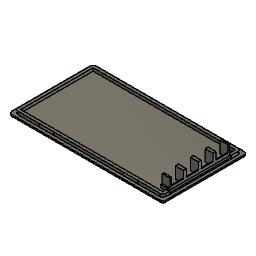
ROC_rev_C+_bottom (Autodesk Fusion 360 design; units mm, degrees)
Autodesk Fusion 360 part; units mm, degrees
sketch "Sketch11" plane through (0, 16, 0) normal (0, -1, 0) x (1, 0, 0)
  line L0 (26.9, -42.9) -> (26.9, -57.9)
  arc A0 (24.9, -59.9) -> (26.9, -57.9) centre (24.9, -57.9) ccw
  line L1 (24.9, -59.9) -> (-24.9, -59.9)
  arc A1 (-26.9, -57.9) -> (-24.9, -59.9) centre (-24.9, -57.9) ccw
  line L2 (-26.9, -57.9) -> (-26.9, -42.9)
  line L3 (-26.9, -42.9) -> (-26.9, -32.9)
  line L4 (-26.9, -32.9) -> (-26.9, 14.9)
  line L5 (-26.9, 14.9) -> (-26.9, 24.9)
  line L6 (-26.9, 24.9) -> (-26.9, 39.9)
  arc A2 (-24.9, 41.9) -> (-26.9, 39.9) centre (-24.9, 39.9) ccw
  line L7 (-24.9, 41.9) -> (24.9, 41.9)
  arc A3 (26.9, 39.9) -> (24.9, 41.9) centre (24.9, 39.9) ccw
  line L8 (26.9, 39.9) -> (26.9, 24.9)
  line L9 (26.9, 24.9) -> (26.9, 14.9)
  line L10 (26.9, 14.9) -> (26.9, -32.9)
  line L11 (26.9, -32.9) -> (26.9, -42.9)
  arc A4 (29, 42) -> (27, 44) centre (27, 42) ccw
  line L12 (27, 44) -> (-27, 44)
  arc A5 (-27, 44) -> (-29, 42) centre (-27, 42) ccw
  line L13 (-29, 42) -> (-29, -60)
  arc A6 (-29, -60) -> (-27, -62) centre (-27, -60) ccw
  line L14 (-27, -62) -> (27, -62)
  arc A7 (27, -62) -> (29, -60) centre (27, -60) ccw
  line L15 (29, -60) -> (29, 42)
  line L16 (-26.9, -32.9) -> (-29, -32.9)
  line L17 (-29, -32.9) -> (-29, -42.9)
  line L18 (-29, -42.9) -> (-26.9, -42.9)
  line L19 (-26.9, -42.9) -> (-26.9, -32.9)
  line L20 (-26.9, 24.9) -> (-29, 24.9)
  line L21 (-29, 24.9) -> (-29, 14.9)
  line L22 (-29, 14.9) -> (-26.9, 14.9)
  line L23 (-26.9, 14.9) -> (-26.9, 24.9)
  line L24 (26.9, 24.9) -> (29, 24.9)
  line L25 (29, 24.9) -> (29, 14.9)
  line L26 (29, 14.9) -> (26.9, 14.9)
  line L27 (26.9, 14.9) -> (26.9, 24.9)
  line L28 (26.9, -32.9) -> (29, -32.9)
  line L29 (29, -32.9) -> (29, -42.9)
  line L30 (29, -42.9) -> (26.9, -42.9)
  line L31 (26.9, -42.9) -> (26.9, -32.9)
  dimension "d1" = 10
  dimension "d2" = 2.1
  dimension "d3" = 10
  dimension "d4" = 10
  dimension "d5" = 10
  constraint horizontal L16
  constraint vertical L17
  constraint horizontal L18
  constraint vertical L19
  constraint coincident L3.end L4.start
  constraint horizontal L20
  constraint vertical L21
  constraint horizontal L22
  constraint vertical L23
  constraint coincident L5.end L6.start
  constraint horizontal L24
  constraint vertical L25
  constraint horizontal L26
  constraint vertical L27
  constraint coincident L8.end L9.start
  constraint horizontal L28
  constraint vertical L29
  constraint horizontal L30
  constraint vertical L31
  constraint coincident L10.end L11.start
  measures "d1" distance of L3.end L2.end
  measures "d2" distance of L5.end L20.end
  measures "d3" distance of L5.end L4.end
  measures "d4" distance of L8.end L9.end
  measures "d5" distance of L10.end L0.start
sketch "Sketch2" plane through (0, 0, 0) normal (0, 1, 0) x (1, 0, 0)
  line L0 (51, -29) -> (-51, -29)
  line L1 (-53, -27) -> (-53, 27)
  line L2 (-51, 29) -> (51, 29)
  line L3 (53, 27) -> (53, -27)
  line L4 (53, -29) -> (-53, 29) construction
  line L5 (-53, -29) -> (53, 29) construction
  arc A0 (-51, 29) -> (-53, 27) centre (-51, 27) ccw
  arc A1 (53, 27) -> (51, 29) centre (51, 27) ccw
  arc A2 (51, -29) -> (53, -27) centre (51, -27) ccw
  arc A3 (-53, -27) -> (-51, -29) centre (-51, -27) ccw
  dimension "d255" = 106
  dimension "d256" = 58
  dimension "d257" = 2
  dimension "d265" = 0
  dimension "d266" = 0
  dimension "d267" = 0
  dimension "d268" = 0
  constraint perpendicular L0 L1
  constraint parallel L0 L2
  constraint parallel L1 L3
  constraint horizontal L0
  constraint coincident L4 origin
  constraint coincident L5 origin
  constraint coincident L4.end L1
  constraint coincident L4.end L2
  constraint tangent L1 A0
  constraint tangent L2 A0
  constraint coincident L5.end L2
  constraint coincident L5.end L3
  constraint tangent L2 A1
  constraint tangent L3 A1
  constraint equal A0 A1
  constraint coincident L4.start L3
  constraint coincident L4.start L0
  constraint tangent L3 A2
  constraint tangent L0 A2
  constraint equal A0 A2
  constraint coincident L5.start L0
  constraint coincident L5.start L1
  constraint tangent L0 A3
  constraint tangent L1 A3
  constraint equal A0 A3
  measures "d255" distance of L4.end L5.end
  measures "d256" distance of L5.start L4.end
  measures "d257" radius of A0
extrude "Extrude1" add sketch "Sketch2" along normal blind 2
sketch "Sketch3" plane through (0, 2, 0) normal (0, 1, 0) x (-1, 0, 0)
  arc A0 (51, -29) -> (53, -27) centre (51, -27) ccw
  line L0 (53, -27) -> (53, 27)
  arc A1 (53, 27) -> (51, 29) centre (51, 27) ccw
  line L1 (51, 29) -> (-51, 29)
  arc A2 (-51, 29) -> (-53, 27) centre (-51, 27) ccw
  line L2 (-53, 27) -> (-53, -27)
  arc A3 (-53, -27) -> (-51, -29) centre (-51, -27) ccw
  line L3 (-51, -29) -> (51, -29)
  line L4 (50.9, -24.9) -> (50.9, 24.9)
  line L5 (48.9, 26.9) -> (-48.9, 26.9)
  line L6 (-50.9, 24.9) -> (-50.9, -24.9)
  line L7 (-48.9, -26.9) -> (48.9, -26.9)
  arc A4 (48.9, -26.9) -> (50.9, -24.9) centre (48.9, -24.9) ccw
  arc A5 (-50.9, -24.9) -> (-48.9, -26.9) centre (-48.9, -24.9) ccw
  arc A6 (-48.9, 26.9) -> (-50.9, 24.9) centre (-48.9, 24.9) ccw
  arc A7 (50.9, 24.9) -> (48.9, 26.9) centre (48.9, 24.9) ccw
  line L8 (-48.9, 24.9) -> (-48.9, -24.9)
  line L9 (-48.9, -24.9) -> (48.9, -24.9)
  line L10 (48.9, -24.9) -> (48.9, 24.9)
  line L11 (48.9, 24.9) -> (-48.9, 24.9)
  dimension "d261" = 2
  dimension "d262" = -2
  dimension "d277" = 2.1
  dimension "d278" = 2.1
  dimension "d279" = 2.1
  dimension "d280" = 2.1
  constraint parallel L0 L4
  constraint parallel L1 L5
  constraint parallel L2 L6
  constraint parallel L3 L7
  constraint tangent L4 A4
  constraint tangent L7 A4
  constraint tangent L7 A5
  constraint tangent L6 A5
  constraint equal A4 A5
  constraint tangent L5 A6
  constraint tangent L6 A6
  constraint equal A4 A6
  constraint tangent L5 A7
  constraint tangent L4 A7
  constraint equal A4 A7
  measures "d261" radius of A4
  measures "d277" distance of L3 L7
  measures "d278" distance of L0 L4
  measures "d279" distance of L1 L5
  measures "d280" distance of L2 L6
extrude "Extrude2" add sketch "Sketch3" along normal blind 2 contours L4 L5 L6 L7 A4 A5 A6 A7
sketch "Sketch4" plane through (0, 0, 26.9) normal (0, 0, 1) x (1, 0, 0)
  line L0 (-48.9, 2) -> (48.9, 2)
  line L1 (48.9, 2) -> (48.9, 4)
  line L2 (48.9, 4) -> (-48.9, 4)
  line L3 (-48.9, 4) -> (-48.9, 2)
  line L4 (33.9, 4) -> (23.9, 4)
  line L5 (23.9, 4) -> (23.9, 2)
  line L6 (23.9, 2) -> (33.9, 2)
  line L7 (33.9, 2) -> (33.9, 4)
  line L8 (-23.9, 4) -> (-33.9, 4)
  line L9 (-33.9, 4) -> (-33.9, 2)
  line L10 (-33.9, 2) -> (-23.9, 2)
  line L11 (-23.9, 2) -> (-23.9, 4)
  dimension "d289" = 10
  dimension "d290" = 10
  dimension "d291" = 15
  dimension "d292" = 15
  constraint horizontal L4
  constraint vertical L5
  constraint horizontal L6
  constraint vertical L7
  constraint coincident L2 L4.start
  constraint horizontal L8
  constraint vertical L9
  constraint horizontal L10
  constraint vertical L11
  constraint coincident L2 L8.start
  measures "d289" distance of L4.start L4.end
  measures "d290" distance of L8.start L8.end
  measures "d291" distance of L3 L9
  measures "d292" distance of L1 L7
extrude "Extrude3" add sketch "Sketch4" along normal blind 1 contours L0 L2 L8 L9 L10 L11 | L0 L2 L4 L5 L6 L7
sketch "Sketch5" plane through (-33.9, 0, 0) normal (-1, 0, 0) x (0, 0, 1)
  line L0 (26.9, 4) -> (26.9, 2)
  line L1 (26.9, 2) -> (27.9, 2)
  line L2 (27.9, 2) -> (27.9, 4)
  line L3 (27.9, 4) -> (26.9, 4)
  line L4 (26.9, 4) -> (27.9, 3)
  line L5 (26.9, 2) -> (27.9, 3)
  constraint coincident L0.start L3.end
  constraint midpoint L2 L4.end
  constraint coincident L0.end L1.start
extrude "Extrude4" cut sketch "Sketch5" against normal up to surface (67.8 mm away) contours L2 L3 L4 | L1 L2 L5
sketch "Sketch6" plane through (0, 0, -26.9) normal (0, 0, -1) x (-1, 0, 0)
  line L0 (-48.9, 2) -> (48.9, 2)
  line L1 (48.9, 2) -> (48.9, 4)
  line L2 (48.9, 4) -> (-48.9, 4)
  line L3 (-48.9, 4) -> (-48.9, 2)
  line L4 (33.9, 4) -> (23.9, 4)
  line L5 (23.9, 4) -> (23.9, 2)
  line L6 (23.9, 2) -> (33.9, 2)
  line L7 (33.9, 2) -> (33.9, 4)
  line L8 (-23.9, 4) -> (-33.9, 4)
  line L9 (-33.9, 4) -> (-33.9, 2)
  line L10 (-33.9, 2) -> (-23.9, 2)
  line L11 (-23.9, 2) -> (-23.9, 4)
  dimension "d297" = 10
  dimension "d298" = 10
  dimension "d299" = 15
  dimension "d300" = 15
  constraint horizontal L4
  constraint vertical L5
  constraint horizontal L6
  constraint vertical L7
  constraint coincident L2 L4.start
  constraint horizontal L8
  constraint vertical L9
  constraint horizontal L10
  constraint vertical L11
  constraint coincident L2 L8.start
  measures "d297" distance of L4.start L4.end
  measures "d298" distance of L8.start L8.end
  measures "d299" distance of L1 L7
  measures "d300" distance of L3 L9
extrude "Extrude5" add sketch "Sketch6" along normal blind 1 contours L0 L2 L8 L9 L10 L11 | L0 L2 L4 L5 L6 L7
sketch "Sketch7" plane through (33.9, 0, 0) normal (1, 0, 0) x (0, 0, -1)
  line L0 (26.9, 4) -> (26.9, 2)
  line L1 (26.9, 2) -> (27.9, 2)
  line L2 (27.9, 2) -> (27.9, 4)
  line L3 (27.9, 4) -> (26.9, 4)
  line L4 (26.9, 4) -> (27.9, 3)
  line L5 (27.9, 3) -> (26.9, 2)
  constraint coincident L0.start L3.end
  constraint midpoint L2 L4.end
  constraint coincident L0.end L1.start
extrude "Extrude6" cut sketch "Sketch7" against normal up to surface (67.8 mm away) contours L2 L3 L4 | L1 L2 L5
extrude "Extrude7" cut sketch "Sketch11" against normal blind 1 contours L11 L15 L28 L29 L30 L31 | L9 L15 L24 L25 L26 L27 | L3 L13 L16 L17 L18 L19 | L5 L13 L20 L21 L22 L23
chamfer "Chamfer1" [no effect]
fillet "Fillet1" radius 0.1 4 edges at (-28.9, 3, 27.9) (28.9, 3, 27.9) (-28.9, 3, -27.9) (28.9, 3, -27.9)
fillet "Fillet2" radius 1 8 edges at (-52.4142, 0, 28.4142) (-53, 0, 0) (-52.4142, 0, -28.4142) (0, 0, -29) (52.4142, 0, -28.4142) (53, 0, 0) (52.4142, 0, 28.4142) (0, 0, 29)
sketch "Sketch8" plane through (0, 2, 0) normal (0, 1, 0) x (-1, 0, 0)
  line L0 (-48.9, 24.9) -> (-48.9, -24.9)
  line L1 (-48.9, -24.9) -> (48.9, -24.9)
  line L2 (48.9, -24.9) -> (48.9, 24.9)
  line L3 (48.9, 24.9) -> (-48.9, 24.9)
  line L4 (-48.9, 21.4) -> (-43.9, 21.4)
  line L5 (-43.9, 21.4) -> (-43.9, 19.4)
  line L6 (-43.9, 19.4) -> (-48.9, 19.4)
  line L7 (-48.9, 19.4) -> (-48.9, 21.4)
  line L8 (-48.9, 24.9) -> (48.9, 24.9)
  line L9 (-48.9, 11.2) -> (-43.9, 11.2)
  line L10 (-43.9, 11.2) -> (-43.9, 9.2)
  line L11 (-43.9, 9.2) -> (-48.9, 9.2)
  line L12 (-48.9, 9.2) -> (-48.9, 11.2)
  line L13 (-48.9, 1) -> (-43.9, 1)
  line L14 (-43.9, 1) -> (-43.9, -1)
  line L15 (-43.9, -1) -> (-48.9, -1)
  line L16 (-48.9, -1) -> (-48.9, 1)
  line L17 (-48.9, -9.2) -> (-43.9, -9.2)
  line L18 (-43.9, -9.2) -> (-43.9, -11.2)
  line L19 (-43.9, -11.2) -> (-48.9, -11.2)
  line L20 (-48.9, -11.2) -> (-48.9, -9.2)
  line L21 (-48.9, -19.4) -> (-43.9, -19.4)
  line L22 (-43.9, -19.4) -> (-43.9, -21.4)
  line L23 (-43.9, -21.4) -> (-48.9, -21.4)
  line L24 (-48.9, -21.4) -> (-48.9, -19.4)
  dimension "d281" = 0
  dimension "d282" = 0
  dimension "d283" = 0
  dimension "d284" = 0
  dimension "d368" = 5
  dimension "d369" = 2
  dimension "d370" = 3.5
  dimension "d375" = 2
  dimension "d376" = 5
  dimension "d377" = 8.2
  dimension "d378" = 2
  dimension "d379" = 5
  dimension "d380" = 5
  dimension "d381" = 2
  dimension "d382" = 8.2
  dimension "d383" = 8.2
  dimension "d384" = 5
  dimension "d385" = 2
  dimension "d386" = 8.2
  constraint horizontal L4
  constraint vertical L5
  constraint horizontal L6
  constraint vertical L7
  constraint coincident L0 L4.start
  constraint horizontal L9
  constraint vertical L10
  constraint horizontal L11
  constraint vertical L12
  constraint coincident L0 L9.start
  constraint horizontal L13
  constraint vertical L14
  constraint horizontal L15
  constraint vertical L16
  constraint coincident L0 L13.start
  constraint horizontal L17
  constraint vertical L18
  constraint horizontal L19
  constraint vertical L20
  constraint coincident L0 L17.start
  constraint horizontal L21
  constraint vertical L22
  constraint horizontal L23
  constraint vertical L24
  constraint coincident L0 L21.start
  measures "d368" distance of L4.start L4.end
  measures "d369" distance of L4.start L6.end
  measures "d370" distance of L4 L8
  measures "d375" distance of L9.start L11.end
  measures "d376" distance of L9.start L9.end
  measures "d377" distance of L6 L9
  measures "d378" distance of L13.start L15.end
  measures "d379" distance of L13.start L13.end
  measures "d380" distance of L17.start L17.end
  measures "d381" distance of L17.start L19.end
  measures "d382" distance of L11 L13
  measures "d383" distance of L15 L17
  measures "d384" distance of L21.start L21.end
  measures "d385" distance of L21.start L23.end
  measures "d386" distance of L19 L21
extrude "Extrude8" add sketch "Sketch8" along normal up to surface (2 mm away) contours L0 L4 L5 L6 L7 | L0 L9 L10 L11 L12 | L0 L21 L22 L23 L24 | L0 L13 L14 L15 L16 | L0 L17 L18 L19 L20
sketch "Sketch9" plane through (0, 4, 0) normal (0, 1, 0) x (-1, 0, 0)
  line L0 (-48.9, 24.9) -> (48.9, 24.9)
  line L1 (48.9, 24.9) -> (48.9, -24.9)
  line L2 (48.9, -24.9) -> (-48.9, -24.9)
  line L3 (-48.9, -24.9) -> (-48.9, -21.4)
  line L4 (-48.9, 19.4) -> (-43.9, 19.4)
  line L5 (-43.9, 19.4) -> (-43.9, 21.4)
  line L6 (-43.9, 21.4) -> (-48.9, 21.4)
  line L7 (-48.9, 21.4) -> (-48.9, 24.9)
  line L8 (-33.9, -26.9) -> (-23.9, -26.9)
  line L9 (-23.9, -26.9) -> (23.9, -26.9)
  line L10 (23.9, -26.9) -> (33.9, -26.9)
  line L11 (33.9, -26.9) -> (48.9, -26.9)
  arc A0 (48.9, -26.9) -> (50.9, -24.9) centre (48.9, -24.9) ccw
  line L12 (50.9, -24.9) -> (50.9, 24.9)
  arc A1 (50.9, 24.9) -> (48.9, 26.9) centre (48.9, 24.9) ccw
  line L13 (48.9, 26.9) -> (33.9, 26.9)
  line L14 (33.9, 26.9) -> (23.9, 26.9)
  line L15 (23.9, 26.9) -> (-23.9, 26.9)
  line L16 (-23.9, 26.9) -> (-33.9, 26.9)
  line L17 (-33.9, 26.9) -> (-48.9, 26.9)
  arc A2 (-48.9, 26.9) -> (-50.9, 24.9) centre (-48.9, 24.9) ccw
  line L18 (-50.9, 24.9) -> (-50.9, -24.9)
  arc A3 (-50.9, -24.9) -> (-48.9, -26.9) centre (-48.9, -24.9) ccw
  line L19 (-48.9, -26.9) -> (-33.9, -26.9)
  line L20 (-48.9, -21.4) -> (-43.9, -21.4)
  line L21 (-43.9, -21.4) -> (-43.9, -19.4)
  line L22 (-43.9, -19.4) -> (-48.9, -19.4)
  line L23 (-48.9, -19.4) -> (-48.9, -11.2)
  line L24 (-48.9, -11.2) -> (-43.9, -11.2)
  line L25 (-43.9, -11.2) -> (-43.9, -9.2)
  line L26 (-43.9, -9.2) -> (-48.9, -9.2)
  line L27 (-48.9, -9.2) -> (-48.9, -1)
  line L28 (-48.9, -1) -> (-43.9, -1)
  line L29 (-43.9, -1) -> (-43.9, 1)
  line L30 (-43.9, 1) -> (-48.9, 1)
  line L31 (-48.9, 1) -> (-48.9, 9.2)
  line L32 (-48.9, 9.2) -> (-43.9, 9.2)
  line L33 (-43.9, 9.2) -> (-43.9, 11.2)
  line L34 (-43.9, 11.2) -> (-48.9, 11.2)
  line L35 (-48.9, 11.2) -> (-48.9, 19.4)
  line L36 (-43.9, -9.2) -> (-50.9, -9.2)
  line L37 (-50.9, -9.2) -> (-50.9, -11.2)
  line L38 (-50.9, -11.2) -> (-43.9, -11.2)
  line L39 (-43.9, -11.2) -> (-43.9, -9.2)
  line L40 (-43.9, 1) -> (-50.9, 1)
  line L41 (-50.9, 1) -> (-50.9, -1)
  line L42 (-50.9, -1) -> (-43.9, -1)
  line L43 (-43.9, -1) -> (-43.9, 1)
  line L44 (-43.9, 11.2) -> (-50.9, 11.2)
  line L45 (-50.9, 11.2) -> (-50.9, 9.2)
  line L46 (-50.9, 9.2) -> (-43.9, 9.2)
  line L47 (-43.9, 9.2) -> (-43.9, 11.2)
  line L48 (-43.9, -19.4) -> (-50.9, -19.4)
  line L49 (-50.9, -19.4) -> (-50.9, -20.4)
  line L50 (-50.9, -20.4) -> (-43.9, -20.4)
  line L51 (-43.9, -20.4) -> (-43.9, -19.4)
  line L52 (-43.9, 19.4) -> (-50.9, 19.4)
  line L53 (-50.9, 19.4) -> (-50.9, 20.4)
  line L54 (-50.9, 20.4) -> (-43.9, 20.4)
  line L55 (-43.9, 20.4) -> (-43.9, 19.4)
  dimension "d389" = 7
  dimension "d390" = 2
  dimension "d393" = 7
  dimension "d394" = 2
  dimension "d397" = 7
  dimension "d398" = 2
  dimension "d401" = 7
  dimension "d402" = 1
  dimension "d403" = 1
  dimension "d404" = 7
  constraint horizontal L36
  constraint vertical L37
  constraint horizontal L38
  constraint vertical L39
  constraint coincident L25.end L26.start
  constraint horizontal L40
  constraint vertical L41
  constraint horizontal L42
  constraint vertical L43
  constraint coincident L29.end L30.start
  constraint horizontal L44
  constraint vertical L45
  constraint horizontal L46
  constraint vertical L47
  constraint coincident L33.end L34.start
  constraint horizontal L48
  constraint vertical L49
  constraint horizontal L50
  constraint vertical L51
  constraint coincident L21.end L22.start
  constraint horizontal L52
  constraint vertical L53
  constraint horizontal L54
  constraint vertical L55
  constraint coincident L4.end L5.start
  measures "d389" distance of L25.end L36.end
  measures "d390" distance of L25.end L24.end
  measures "d393" distance of L29.end L40.end
  measures "d394" distance of L29.end L28.end
  measures "d397" distance of L33.end L44.end
  measures "d398" distance of L33.end L32.end
  measures "d401" distance of L21.end L48.end
  measures "d402" distance of L21.end L50.end
  measures "d403" distance of L4.end L54.end
  measures "d404" distance of L4.end L52.end
extrude "Extrude9" add sketch "Sketch9" along normal blind 6 contours L4 L5 L18 L52 L53 L54 L55 | L18 L21 L22 L48 L49 L50 L51 | L18 L32 L33 L34 L44 L45 L46 L47 | L18 L28 L29 L30 L40 L41 L42 L43 | L18 L24 L25 L26 L36 L37 L38 L39
extrude "Extrude10" add 4 faces at (50.2333, 4, 13.9333) (50.2333, 4, 6.4667) (50.2333, 4, -6.4667) (50.2333, 4, -13.9333) along direction (0, 1, 0) blind 1
sketch "Sketch10" plane through (50.9, 0, 0) normal (1, 0, 0) x (0, 0, -1)
  line L0 (-24.9, 2) -> (24.9, 2)
  line L1 (24.9, 2) -> (24.9, 4)
  line L2 (20.4, 10) -> (19.4, 10)
  line L3 (19.4, 10) -> (19.4, 5)
  line L4 (19.4, 5) -> (11.2, 5)
  line L5 (11.2, 5) -> (11.2, 10)
  line L6 (11.2, 10) -> (9.2, 10)
  line L7 (9.2, 10) -> (9.2, 5)
  line L8 (9.2, 5) -> (1, 5)
  line L9 (1, 5) -> (1, 10)
  line L10 (1, 10) -> (-1, 10)
  line L11 (-1, 10) -> (-1, 5)
  line L12 (-24.9, 4) -> (-24.9, 2)
  line L13 (20.4, 10) -> (-22.4, 10)
  line L14 (-22.4, 10) -> (-22.4, 3)
  line L15 (-22.4, 3) -> (20.4, 3)
  line L16 (20.4, 3) -> (20.4, 10)
  line L17 (-20.4, 10) -> (-20.4, 4)
  line L18 (24.9, 4) -> (20.4, 4)
  line L19 (20.4, 4) -> (20.4, 10)
  line L20 (-11.2, 5) -> (-19.4, 5)
  line L21 (-19.4, 5) -> (-19.4, 10)
  line L22 (-19.4, 10) -> (-20.4, 10)
  line L23 (-1, 5) -> (-9.2, 5)
  line L24 (-9.2, 5) -> (-9.2, 10)
  line L25 (-9.2, 10) -> (-11.2, 10)
  line L26 (-11.2, 10) -> (-11.2, 5)
  line L27 (-20.4, 4) -> (-24.9, 4)
  constraint horizontal L13
  constraint vertical L14
  constraint horizontal L15
  constraint vertical L16
  constraint coincident L2.start L13.start
extrude "Extrude11" cut sketch "Sketch10" against normal blind 1.5 contours L2 L3 L4 L5 L6 L7 L8 L9 L10 L11 L13 L14 L15 L16 L17 L19 L20 L21 L22 L23 L24 L25 L26 L27 | L13 L14 L17 L27 | L13 L20 L21 L26 | L11 L13 L23 L24
equation "d382 = d377"
equation "d383 = d377"
equation "d386 = d377"
